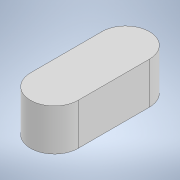
# Autodesk Inventor part: CHAVETA UNE 17012 8X7X20
Saved by Autodesk Inventor 2020 (Build 240168000, 168)
## iProperties
Created: 2021-01-08
Part Number: CHAVETA UNE 17012 8X7X20
Material: Genérico
Document SubType Name: Chapa
Designer: equipo-pcfactory
Density: 1 g/cm^3
Sheet Metal Rule: Por defecto_mm
Appearance: Valor por defecto
Author: equipo-pcfactory
Autodesk Inventor part; units mm, degrees
ref_plane "YZ Plane" through (0, 0, 0) normal (1, 0, 0) x (0, 1, 0)
ref_plane "XZ Plane" through (0, 0, 0) normal (0, 1, 0) x (-1, 0, 0)
ref_plane "XY Plane" through (0, 0, 0) normal (0, 0, 1) x (1, 0, 0)
sketch "Boceto1" plane through (0, 0, 0) normal (0, 1, 0) x (-1, 0, 0)
  circle A0 centre (0, 0) radius 4
  line L0 (0, 4) -> (0, -16)
  line L1 (0, -16) -> (0, -12)
  circle A1 centre (0, -12) radius 4
  line L2 (4, 0) -> (4, -12)
  line L3 (-4, 0) -> (-4, -12)
  dimension "d0" = 8
  dimension "d1" = 20
  dimension "d2" = 4
  dimension "d3" = 8
  constraints: 8 end point, 5 point on circle, 2 centre point, 2 coincident, 2 tangent, 1 point on line, 1 vertical
  measures "d0" diameter of A0
  measures "d1" distance of L0.start L0.end
  measures "d2" distance of L0.end L1.end
  measures "d3" diameter of A1
extrude "Extrusión1" add sketch "Boceto1" along normal blind 7
equation "\"Radio_pliegue\" = Grosor"
equation "\"Anchura_desahogo_plegado\" = Grosor"
equation "\"Profundidad_desahogo_plegado\" = 0.5 * Grosor"
equation "\"Tamaño_destalonado\" = 4 * Grosor"
equation "\"Remanente_mínimo\" = 2 * Grosor"
equation "\"Radiodetransición\" = Radio_pliegue"
equation "\"Tamaño_de_radio_de_Jacobi\" = Radio_pliegue"
equation "\"TamañoSeparación\" = Grosor"
equation "\"Grosor\" = 0.5"
